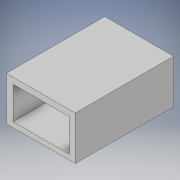
# Autodesk Inventor part: connection
Saved by Autodesk Inventor 2019 (Build 230136000, 136)
## iProperties
Created: 2019-12-08
Part Number: connection
Material: Generic
Document SubType Name: Modeling
Designer: HP
Density: 1 g/cm^3
Appearance: Default
Author: HP
Autodesk Inventor part; units mm, degrees
ref_plane "YZ Plane" through (0, 0, 0) normal (1, 0, 0) x (0, 1, 0)
ref_plane "XZ Plane" through (0, 0, 0) normal (0, 1, 0) x (-1, 0, 0)
ref_plane "XY Plane" through (0, 0, 0) normal (0, 0, 1) x (1, 0, 0)
sketch "Sketch1" plane through (0, 0, 0) normal (0, 0, 1) x (1, 0, 0)
  line L0 (0, 0) -> (7.112, 0)
  line L1 (7.112, 0) -> (7.112, 4.5212)
  line L2 (7.112, 4.5212) -> (0, 4.5212)
  line L3 (0, 4.5212) -> (0, 0)
  dimension "d0" = 7.112
  dimension "d1" = 4.5212
  constraints: 8 end point, 2 parallel, 1 horizontal, 1 perpendicular
  measures "d0" distance of L2.end L1.end
  measures "d1" distance of L1.end L0.end
extrude "Extrusion1" add sketch "Sketch1" along normal blind 10.16
sketch "Sketch2" plane through (0, 0, 10.16) normal (0, 0, 1) x (1, 0, 0)
  line L0 (0.6954, 3.8901) -> (6.5198, 3.8901)
  line L1 (6.5198, 3.8901) -> (6.5198, 0.5433)
  line L2 (6.5198, 0.5433) -> (0.6954, 0.5433)
  line L3 (0.6954, 0.5433) -> (0.6954, 3.8901)
  point P0 (0, 0)
  constraints: 8 end point, 2 parallel, 1 horizontal, 1 perpendicular
extrude "Extrusion2" cut sketch "Sketch2" against normal blind 10.16
body "Solid1"
